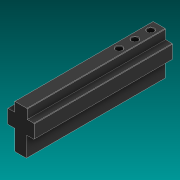
# Autodesk Inventor part: slider
Saved by Autodesk Inventor 2020.3 (Build 243373000, 373)
## iProperties
Created: 2020-05-25
Part Number: slider
Material: Generic
Document SubType Name: Modeling
Designer: Svend
Density: 1 g/cm^3
Appearance: Default
Author: Svend
Autodesk Inventor part; units mm, degrees
ref_plane "YZ Plane" through (0, 0, 0) normal (1, 0, 0) x (0, 1, 0)
ref_plane "XZ Plane" through (0, 0, 0) normal (0, 1, 0) x (-1, 0, 0)
ref_plane "XY Plane" through (0, 0, 0) normal (0, 0, 1) x (1, 0, 0)
sketch "Sketch1" plane through (0, 0, 0) normal (0, 0, 1) x (1, 0, 0)
  line L0 (-3.25, 4.8) -> (3.25, 4.8)
  line L1 (3.25, 4.8) -> (3.25, 0)
  line L2 (3.25, 0) -> (6.8, 0)
  line L3 (6.8, 0) -> (6.8, -7)
  line L4 (-3, -17.2) -> (-3, -7)
  line L5 (-6.8, -7) -> (-6.8, 0)
  line L6 (-6.8, 0) -> (-3.25, 0)
  line L7 (-3.25, 4.8) -> (-3.25, 0)
  line L8 (-3, -17.2) -> (3, -17.2)
  line L9 (6.8, -7) -> (3, -7)
  line L10 (-6.8, -7) -> (-3, -7)
  line L11 (3, -17.2) -> (3, -7)
  point P0 (0, 0)
  point P1 (0, 4.8)
  point P2 (0, -17.2)
  point P3 (0, -17.2)
  dimension "d0" = 6.5
  dimension "d1" = 4.8
  dimension "d6" = 10.2
  dimension "d7" = 7
  dimension "d8" = 6
  dimension "d9" = 13.6
  constraints: 24 end point, 5 perpendicular, 4 horizontal, 3 equal length, 3 point on line, 2 midpoint, 2 vertical, 2 vertical alignment, 1 coincident
  measures "d0" distance between parallel lines of L7 L1
  measures "d1" distance between parallel lines of L2 L0
  measures "d6" distance of L4.start L4.end
  measures "d7" distance of L2.end L3.end
  measures "d8" distance between parallel lines of L4 L11
  measures "d9" distance between parallel lines of L5 L3
extrude "Extrusion1" add sketch "Sketch1" along normal mid plane 70
sketch "Sketch2" plane through (-3.25, 4.8, 35) normal (0, 1, 0) x (1, 0, 0)
  line L0 (0, 70) -> (0, 0) projected
  line L1 (6.5, 0) -> (0, 0) projected
  line L2 (6.5, 70) -> (6.5, 0) projected
  line L3 (0, 70) -> (6.5, 70) projected
  circle A0 centre (3.25, 49.7) radius 1.6
  circle A1 centre (3.25, 57.7) radius 1.6
  circle A2 centre (3.25, 65.7) radius 1.6
  point P0 (3.25, 35)
  dimension "d13" = 4.3
  dimension "d14" = 8
  dimension "d15" = 8
  dimension "d17" = 3.2
  constraints: 3 centre point, 3 coincident, 3 vertical alignment, 2 equal radius
  measures "d13" distance from line of point (3.25, 65.7) L3
  measures "d14" distance of point (3.25, 57.7) point (3.25, 65.7)
  measures "d15" distance of point (3.25, 57.7) point (3.25, 49.7)
  measures "d17" diameter of A0
extrude "Extrusion2" cut sketch "Sketch2" against normal blind 8.3 contours A0 | A1 | A2
sketch "Sketch3" plane through (0, 0, -35) normal (0, 0, -1) x (-1, 0, 0)
  line L0 (3, -17.2) -> (3, -7) projected
  line L1 (3, -7) -> (6.8, -7) projected
  line L2 (6.8, -7) -> (6.8, 0) projected
  line L3 (6.8, 0) -> (3.25, 0) projected
  line L4 (3.25, 0) -> (3.25, 4.8) projected
  line L5 (3.25, 4.8) -> (-3.25, 4.8) projected
  line L6 (-3.25, 4.8) -> (-3.25, 0) projected
  line L7 (-3.25, 0) -> (-6.8, 0) projected
  line L8 (-6.8, 0) -> (-6.8, -7) projected
  line L9 (-6.8, -7) -> (-3, -7) projected
  line L10 (-3, -7) -> (-3, -17.2) projected
  line L11 (-3, -17.2) -> (3, -17.2) projected
  line L12 (-1.6, -3.5) -> (1.6, -3.5) projected
  line L13 (-2.75, -1.5) -> (2.75, -1.5)
  line L14 (2.75, -1.5) -> (2.75, -5.5)
  line L15 (2.75, -5.5) -> (-2.75, -5.5)
  line L16 (-2.75, -5.5) -> (-2.75, -1.5)
  line L17 (-2.75, -1.5) -> (2.75, -5.5) construction
  line L18 (2.75, -1.5) -> (-2.75, -5.5) construction
  point P0 (0, 0)
  point P1 (0, -3.5)
  dimension "d21" = 5.5
  dimension "d22" = 4
  constraints: 12 end point, 3 midpoint, 2 parallel, 1 horizontal, 1 perpendicular
  measures "d21" distance of L14.end L15.end
  measures "d22" distance of L13.end L14.end
extrude "Extrusion3" cut sketch "Sketch3" against normal blind 25 contours L13 L14 L15 L16
chamfer "Chamfer1" distance 0.2 angle 45 8 edges at (6.8, 0, 0) (6.8, -7, 0) (3.25, 4.8, 0) (-3.25, 4.8, 0) (-6.8, 0, 0) (-6.8, -7, 0) (-3, -17.2, 0) (3, -17.2, 0)
chamfer "Chamfer2" distance 0.2 angle 45 3 edges at (-1.6, 4.8, -14.7) (-1.6, 4.8, -22.7) (-1.6, 4.8, -30.7)
equation "\"d15\" = d14"
body "Solid1"
